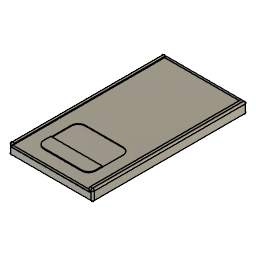
Small Drill Bit Box v3 (Autodesk Fusion 360 design; units mm, degrees)
Autodesk Fusion 360 part; units mm, degrees
sketch "Sketch1" plane through (0, 0, 0) normal (0, 0, 1) x (1, 0, 0)
  line L0 (24.2, 3) -> (14.2, 3)
  line L1 (14.2, 3) -> (14.2, 68)
  line L2 (14.2, 68) -> (24.2, 68)
  line L3 (24.2, 68) -> (24.2, 3)
  line L4 (24.2, 3) -> (14.2, 68) construction
  line L5 (14.2, 3) -> (24.2, 68) construction
  line L6 (35.4, 3) -> (25.4, 3)
  line L7 (25.4, 3) -> (25.4, 55.5)
  line L8 (25.4, 55.5) -> (35.4, 55.5)
  line L9 (35.4, 55.5) -> (35.4, 3)
  line L10 (35.4, 3) -> (25.4, 55.5) construction
  line L11 (25.4, 3) -> (35.4, 55.5) construction
  line L12 (24.2, 69.2) -> (14.2, 69.2)
  line L13 (14.2, 69.2) -> (14.2, 109.2)
  line L14 (14.2, 109.2) -> (24.2, 109.2)
  line L15 (24.2, 109.2) -> (24.2, 69.2)
  line L16 (24.2, 69.2) -> (14.2, 109.2) construction
  line L17 (14.2, 69.2) -> (24.2, 109.2) construction
  line L18 (35.4, 56.7) -> (25.4, 56.7)
  line L19 (25.4, 56.7) -> (25.4, 109.2)
  line L20 (25.4, 109.2) -> (35.4, 109.2)
  line L21 (35.4, 109.2) -> (35.4, 56.7)
  line L22 (35.4, 56.7) -> (25.4, 109.2) construction
  line L23 (25.4, 56.7) -> (35.4, 109.2) construction
  line L24 (13, 68) -> (13, 3)
  line L25 (13, 3) -> (3, 3)
  line L26 (3, 68) -> (13, 68)
  line L27 (3, 3) -> (3, 68)
  line L28 (3, 109.2) -> (13, 109.2)
  line L29 (13, 109.2) -> (13, 69.2)
  line L30 (3, 69.2) -> (3, 109.2)
  line L31 (13, 69.2) -> (3, 69.2)
  line L32 (36.6, 109.2) -> (46.6, 109.2)
  line L33 (46.6, 109.2) -> (46.6, 56.7)
  line L34 (36.6, 56.7) -> (36.6, 109.2)
  line L35 (46.6, 56.7) -> (36.6, 56.7)
  line L36 (36.6, 55.5) -> (46.6, 55.5)
  line L37 (46.6, 55.5) -> (46.6, 3)
  line L38 (36.6, 3) -> (36.6, 55.5)
  line L39 (46.6, 3) -> (36.6, 3)
  line L40 (47.8, 109.2) -> (57.8, 109.2)
  line L41 (57.8, 109.2) -> (57.8, 56.7)
  line L42 (47.8, 56.7) -> (47.8, 109.2)
  line L43 (57.8, 56.7) -> (47.8, 56.7)
  line L44 (47.8, 55.5) -> (57.8, 55.5)
  line L45 (57.8, 55.5) -> (57.8, 3)
  line L46 (47.8, 3) -> (47.8, 55.5)
  line L47 (57.8, 3) -> (47.8, 3)
  line L48 (0, 0) -> (60.8, 0)
  line L49 (60.8, 0) -> (60.8, 112.2)
  line L50 (60.8, 112.2) -> (0, 112.2)
  line L51 (0, 112.2) -> (0, 0)
  point P0 (19.2, 35.5)
  point P1 (30.4, 29.25)
  point P2 (19.2, 89.2)
  point P3 (30.4, 82.95)
  dimension "d48" = 65
  dimension "d50" = 10
  dimension "d51" = 10
  dimension "d52" = 52.5
  dimension "d53" = 10
  dimension "d54" = 40
  dimension "d55" = 1.2
  dimension "d56" = 10
  dimension "d57" = 52.5
  dimension "d58" = 1.2
  dimension "d62" = 0
  dimension "d65" = 11.2
  dimension "d66" = 0
  dimension "d67" = 3
  dimension "d68" = 3
  dimension "d69" = 3
  dimension "d70" = 3
  constraint horizontal L0
  constraint perpendicular L0 L1
  constraint parallel L0 L2
  constraint parallel L1 L3
  constraint coincident L4 P0
  constraint coincident L5 P0
  constraint horizontal L6
  constraint perpendicular L6 L7
  constraint parallel L6 L8
  constraint parallel L7 L9
  constraint coincident L10 P1
  constraint coincident L11 P1
  constraint horizontal L12
  constraint perpendicular L12 L13
  constraint parallel L12 L14
  constraint parallel L13 L15
  constraint coincident L16 P2
  constraint coincident L17 P2
  constraint horizontal L18
  constraint perpendicular L18 L19
  constraint parallel L18 L20
  constraint parallel L19 L21
  constraint coincident L22 P3
  constraint coincident L23 P3
  constraint collinear L0 L6
  constraint collinear L14 L20
  constraint collinear L7 L19
  constraint collinear L1 L13
  constraint horizontal L48
  constraint vertical L49
  constraint horizontal L50
  constraint vertical L51
  constraint coincident L48.start L51.end
  measures "d48" distance of L0.end L1.end
  measures "d50" distance of L0.start L0.end
  measures "d51" distance of L7.end L8.end
  measures "d52" distance of L6.end L7.end
  measures "d53" distance of L13.end L14.end
  measures "d54" distance of L12.end L13.end
  measures "d55" distance of L2 L12
  measures "d56" distance of L19.end L20.end
  measures "d57" distance of L18.end L19.end
  measures "d58" distance of L3 L7
  measures "d67" distance of L25 L48
  measures "d68" distance of L27 L51
  measures "d69" distance of L40 L50
  measures "d70" distance of L41 L49
extrude "Extrude1" add sketch "Sketch1" along normal blind 1 contours L0 L1 L2 L3 | L6 L7 L8 L9 | L12 L13 L14 L15 | L18 L19 L20 L21 | L24 L25 L26 L27 | L28 L29 L30 L31 | L32 L33 L34 L35 | L36 L37 L38 L39 | L40 L41 L42 L43 | L44 L45 L46 L47 | L48 L49 L50 L51 makes body 1
extrude "Extrude2" add sketch "Sketch1" along normal blind 5 from surface at 1 bodies 1
sketch "Sketch2" plane through (0, 0, 0) normal (0, -1, 0) x (1, 0, 0)
  line L0 (0, 0) -> (60.8, 0)
  line L1 (60.8, 0) -> (60.8, 6)
  line L2 (60.8, 6) -> (0, 6)
  line L3 (0, 6) -> (0, 0)
  line L4 (0, 6) -> (0, 8.4)
  line L5 (0, 8.4) -> (3, 8.4)
  line L6 (3, 8.4) -> (3, 8)
  line L7 (3, 8) -> (2, 7)
  line L8 (2, 7) -> (2, 6)
  line L9 (30.4, 6) -> (30.4, 0) construction
  line L10 (30.4, 6.1) -> (30.4, 7.7) construction
  line L11 (30.4, 7.7) -> (2.9, 7.7)
  line L12 (2.9, 7.7) -> (2.1, 6.9)
  line L13 (2.1, 6.9) -> (2.1, 6.1)
  line L14 (2.1, 6.1) -> (30.4, 6.1)
  line L15 (60.8, 6) -> (60.8, 8.4)
  line L16 (57.8, 8.4) -> (57.8, 8)
  line L17 (57.8, 8) -> (58.8, 7)
  line L18 (58.8, 7) -> (58.8, 6)
  line L19 (60.8, 8.4) -> (57.8, 8.4)
  line L20 (57.9, 7.7) -> (58.7, 6.9)
  line L21 (58.7, 6.9) -> (58.7, 6.1)
  line L22 (58.7, 6.1) -> (30.4, 6.1)
  line L23 (30.4, 7.7) -> (57.9, 7.7)
  point P0 (3, 6)
  point P1 (57.8, 6)
  dimension "d78" = 45
  dimension "d83" = 2.4
  dimension "d86" = 1.6
  dimension "d107" = 0.8
  dimension "d108" = 1
  dimension "d109" = 0.1
  dimension "d110" = 0.1
  dimension "d111" = 2
  dimension "d112" = 0.4
  dimension "d113" = 1
  constraint coincident L2.end L3.start
  constraint perpendicular L2 L4
  constraint perpendicular L4 L5
  constraint perpendicular L5 L6
  constraint vertical L8
  constraint coincident L2 L8.end
  constraint midpoint L2 L9.start
  constraint midpoint L0 L9.end
  constraint perpendicular L2 L10
  constraint perpendicular L10 L11
  constraint perpendicular L11 L13
  constraint perpendicular L10 L14
  constraint parallel L7 L12
  constraint collinear L9 L10
  constraint symmetric L2.end L9 L1.end
  constraint symmetric L4.end L9 L15.end
  constraint symmetric L5.end L9 L16.start
  constraint symmetric L6.end L9 L16.end
  constraint symmetric L7.end L9 L17.end
  constraint symmetric L8.end L9 L18.end
  constraint symmetric L9 L10.start L14.end
  constraint symmetric L9 L10.end L11.start
  constraint symmetric L9 L11.end L20.start
  constraint symmetric L9 L12.end L20.end
  constraint symmetric L9 L13.end L21.end
  constraint horizontal L22
  constraint coincident L10.end L11.start
  measures "d78" angle of L2 L7
  measures "d83" distance of L2.end L4.end
  measures "d86" distance of L11 L14
  measures "d107" distance of L12.end L13.end
  measures "d108" distance of L7.end L8.end
  measures "d109" distance of L2 L14
  measures "d110" distance of L8 L13
  measures "d111" distance of L2.end L8.end
  measures "d112" distance of L5.end L6.end
  measures "d113" horizontal distance of L6.end L7.end
extrude "Extrude3" add sketch "Sketch2" against normal up to surface (112.2 mm away) contours L2 L4 L5 L6 L7 L8 | L2 L15 L16 L17 L18 L19 bodies 1
sketch "Sketch3" plane through (0, 112.2, 0) normal (0, 1, 0) x (-1, 0, 0)
  line L0 (-60.8, 0) -> (0, 0)
  line L1 (0, 0) -> (0, 8.4)
  line L2 (0, 8.4) -> (-3, 8.4)
  line L3 (-3, 8.4) -> (-3, 8)
  line L4 (-3, 8) -> (-2, 7)
  line L5 (-2, 7) -> (-2, 6)
  line L6 (-2, 6) -> (-58.8, 6)
  line L7 (-58.8, 6) -> (-58.8, 7)
  line L8 (-58.8, 7) -> (-57.8, 8)
  line L9 (-57.8, 8) -> (-57.8, 8.4)
  line L10 (-57.8, 8.4) -> (-60.8, 8.4)
  line L11 (-60.8, 8.4) -> (-60.8, 0)
  line L12 (-57.8, 8.4) -> (-3, 8.4)
  constraint coincident L9.end L10.start
  constraint coincident L2.end L3.start
extrude "Extrude4" add sketch "Sketch3" against normal blind 1.2 contours L3 L4 L5 L6 L7 L8 L9 L12 bodies 1
copy_body "Body->Comp1" bodies 1 removing the originals makes body 2 in component "Box"
extrude "Extrude1'" add sketch "Sketch2" against normal up to surface (110.2 mm away) separate body contours L11 L12 L13 L14 L20 L21 L22 L23 makes body 3 in component "Lid"
sketch "Sketch1 (2)" plane through (0, 0, 7.7) normal (0, 0, 1) x (-1, 0, 0) in component "Lid"
  line L0 (-57.9, -110.2) -> (-2.9, -110.2)
  line L1 (-2.9, -110.2) -> (-2.9, 0)
  line L2 (-2.9, 0) -> (-57.9, 0)
  line L3 (-57.9, 0) -> (-57.9, -110.2)
  line L4 (-2.9, 0) -> (-57.9, -55.1) construction
  line L5 (-30.4, -27.55) -> (-57.9, 0) construction
  line L6 (-30.4, 0) -> (-44.15, -13.775) construction
  line L7 (-44.15, -13.775) -> (-16.65, -13.775) construction
  line L8 (-16.65, -8.775) -> (-44.15, -8.775)
  arc A0 (-44.15, -8.775) -> (-44.15, -18.775) centre (-44.15, -13.775) ccw
  line L9 (-44.15, -18.775) -> (-16.65, -18.775)
  arc A1 (-16.65, -18.775) -> (-16.65, -8.775) centre (-16.65, -13.775) ccw
  line L10 (-16.65, -13.775) -> (-44.15, -13.775) construction
  line L11 (-49.15, -13.775) -> (-49.15, -33.775)
  arc A2 (-49.15, -33.775) -> (-44.15, -38.775) centre (-44.15, -33.775) ccw
  line L12 (-44.15, -38.775) -> (-16.65, -38.775)
  arc A3 (-16.65, -38.775) -> (-11.65, -33.775) centre (-16.65, -33.775) ccw
  line L13 (-11.65, -33.775) -> (-11.65, -13.775)
  line L14 (-44.15, -18.775) -> (-49.15, -18.775)
  line L15 (-16.65, -18.775) -> (-11.65, -18.775)
  dimension "d97" = 10
  dimension "d98" = 5
  dimension "d99" = 5
  dimension "d100" = 20
  constraint coincident L1.end L2.start
  constraint midpoint L3 L4.end
  constraint midpoint L4 L5.start
  constraint coincident L2.end L3.start
  constraint midpoint L2 L6.start
  constraint midpoint L5 L6.end
  constraint coincident L4 L7.end
  constraint horizontal L7
  constraint tangent L8 A0
  constraint tangent A0 L9
  constraint parallel L8 L9
  constraint tangent L9 A1
  constraint tangent L8 A1
  constraint coincident L6.end L7.start
  constraint parallel L7 L10
  constraint coincident L7.end A1.centre
  constraint coincident A0 L11.start
  constraint parallel L3 L11
  constraint tangent L11 A2
  constraint perpendicular L11 L12
  constraint tangent L12 A3
  constraint coincident A1 L13.end
  constraint tangent A1 L13
  constraint tangent A0 L11
  constraint parallel L11 L13
  constraint tangent A3 L13
  constraint tangent A2 L12
  constraint coincident L11 L14.end
  constraint tangent A0 L14
  constraint coincident L13 L15.end
  constraint tangent A1 L15
  measures "d97" diameter of A0
  measures "d98" radius of A2
  measures "d99" radius of A3
  measures "d100" distance of L9 L12
extrude "Extrude3'" add sketch "Sketch1 (2)" along normal blind 0.6 contours L8 A0 L9 A1 | A1 L13 L15 | A0 L11 L14 bodies 3 in component "Lid"
extrude "Extrude4'" cut sketch "Sketch1 (2)" against normal blind 0.4 contours L9 L11 A2 L12 A3 L13 L14 L15 bodies 3 in component "Lid"
fillet "Fillet1" radius 1.2 13 edges at (30.4, 0, 0) (60.8, 56.1, 0) (30.4, 112.2, 0) (0, 56.1, 0) (0, 0, 4.2) (60.8, 0, 4.2) (60.8, 112.2, 4.2) (0, 112.2, 4.2) (30.4, 112.2, 8.4) (0, 56.1, 8.4) (1.5, 0, 8.4) (59.3, 0, 8.4) (60.8, 56.1, 8.4) on bodies 2 in component "Box"
component "Lid" placed x (1, 0, 0) y (0, 1, 0) z (0, 0, 1) at (0, 0, 0)
component "Box" placed x (1, 0, 0) y (0, 1, 0) z (0, 0, 1) at (0, 0, 0)
equation "Gap = 1.2 mm"
equation "WalPushback = -0.4 mm"
equation "BitLength1 = 65 mm"
equation "BitLength2 = 52.5 mm"
equation "BitLength3 = 40 mm"
equation "d48 = BitLength1"
equation "CompartmentWidth = 10 mm"
equation "d50 = CompartmentWidth"
equation "d51 = CompartmentWidth"
equation "d52 = BitLength2"
equation "d53 = CompartmentWidth"
equation "d54 = BitLength3"
equation "d55 = Gap"
equation "d56 = CompartmentWidth"
equation "d57 = BitLength2"
equation "d58 = Gap"
equation "d61 = -( CompartmentWidth + Gap )"
equation "d65 = CompartmentWidth + Gap"
equation "d67 = EdgeWidth"
equation "d68 = EdgeWidth"
equation "d69 = EdgeWidth"
equation "d70 = EdgeWidth"
equation "EdgeWidth = 3 mm"
